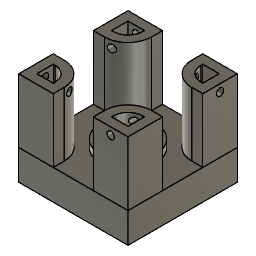
pince (Autodesk Fusion 360 archive; units mm, degrees)
design "pince_v01_structure"
part number: 2026-02-12-14-10-12-234
Autodesk Fusion 360 part; units mm, degrees
sketch "Esquisse1" plane through (0, 0, 0) normal (0, 0, 1) x (1, 0, 0)
  line L0 (30, 30) -> (-30, 30)
  line L1 (-30, 30) -> (-30, -30)
  line L2 (-30, -30) -> (30, -30)
  line L3 (30, -30) -> (30, 30)
  constraint horizontal L0
  constraint vertical L1
  constraint horizontal L2
  constraint vertical L3
extrude "Extrusion1" add sketch "Esquisse1" along normal blind 5 makes body 1
sketch "Esquisse3" plane through (0, 0, 5) normal (0, 0, 1) x (-1, 0, 0)
  line L0 (-30, 30) -> (-30, -30)
  line L1 (-30, -30) -> (30, -30)
  line L2 (30, -30) -> (30, 30)
  line L3 (30, 30) -> (-30, 30)
  circle A0 centre (0, 0) radius 3.5
  circle A1 centre (0, 0) radius 15
  dimension "d12" = 7
  dimension "d15" = 30
  constraint coincident A0.centre A1.centre
  measures "d12" diameter of A0
  measures "d15" diameter of A1
extrude "Extrusion2" add sketch "Esquisse3" along normal blind 4 contours A1 bodies 1
sketch "Esquisse4" plane through (0, 0, 5) normal (0, 0, 1) x (-1, 0, 0)
  line L0 (-30, 30) -> (-30, -30)
  line L1 (-30, -30) -> (30, -30)
  line L2 (30, -30) -> (30, 30)
  line L3 (30, 30) -> (-30, 30)
  circle A0 centre (0, 0) radius 15
  arc A1 (-24, 11) -> (-11, 24) centre (-24, 24) ccw
  line L4 (-11, 24) -> (-30, 24)
  line L5 (-30, 24) -> (-30, 30)
  line L6 (-30, 30) -> (-11, 30)
  line L7 (-11, 30) -> (-11, 24)
  line L8 (-30, 30) -> (-24, 30)
  line L9 (-24, 30) -> (-24, 11)
  line L10 (-24, 11) -> (-30, 11)
  line L11 (-30, 11) -> (-30, 30)
  constraint horizontal L4
  constraint vertical L5
  constraint horizontal L6
  constraint vertical L7
  constraint coincident L0.start L3.end
  constraint horizontal L8
  constraint vertical L9
  constraint horizontal L10
  constraint vertical L11
extrude "Extrusion3" add sketch "Esquisse4" along normal up to surface (70 mm away) contours L0 L3 L4 L5 L6 L8 L9 L11 | L0 L4 L9 L10 L11 | L3 L4 L6 L7 L9 | A1 L4 L9 bodies 1
sketch "Esquisse5" plane through (0, 0, 0) normal (0, 1, 0) x (1, 0, 0)
  line L0 (-30, 0) -> (30, 0)
  line L1 (30, 0) -> (30, 9.0556)
  line L2 (30, 19.372) -> (-30, 19.372)
  line L3 (-30, 9.0556) -> (-30, 0)
  circle A0 centre (0, 36) radius 34.3
  arc A1 (-25.7143, 10.8052) -> (25.7143, 10.8052) centre (0, 36) ccw
  arc A2 (-25.7143, 10.8052) -> (-30, 9.0556) centre (-27.5, 9.0556) ccw
  arc A3 (30, 9.0556) -> (25.7143, 10.8052) centre (27.5, 9.0556) ccw
  line L4 (-30, 7.5) -> (-27.5, 7.5)
  line L5 (-27.5, 7.5) -> (-27.5, 11.5556)
  line L6 (-27.5, 11.5556) -> (-30, 11.5556)
  line L7 (-30, 11.5556) -> (-30, 7.5)
  point P0 (-30, 0)
  dimension "d80" = 36
  dimension "d81" = 2.5
  dimension "d82" = 2.5
  dimension "d83" = 2.5
  constraint horizontal L0
  constraint vertical L1
  constraint horizontal L2
  constraint vertical L3
  constraint coincident L2.start A0
  constraint coincident P0 L0.start
  constraint coincident A0.centre A1.centre
  constraint tangent A1 A2
  constraint tangent L3 A2
  constraint tangent A1 A3
  constraint tangent L1 A3
  constraint horizontal L4
  constraint vertical L5
  constraint horizontal L6
  constraint vertical L7
  constraint coincident L3 L4.start
  measures "d80" radius of A1
  measures "d81" radius of A2
  measures "d82" radius of A3
  measures "d83" distance of L4.start L4.end
revolve "Révolution2" add sketch "Esquisse5" angle 360 about axis through (0, 0, -205.75) along (0, 0, 1) contours L0 L3 A1 A2 L4 L5 | L3 A2 L4 L5 L7 | A2 L6 L7 bodies 1
extrude "Extrusion4" add 4 faces at (-24.1061, -24.1061, 0) (24.1061, -24.1061, 0) (24.1061, 24.1061, 0) (-24.1061, 24.1061, 0) along direction (0, 0, -1) up to surface end surface through (0, 0, -11.5556) normal (0, 0, -1) offset 0 on bodies 1 bodies 1
extrude "Extrusion5" cut 1 faces at (28, -17.3333, 75) along direction (0, 0, -1) blind 35 on bodies 1 bodies 1
sketch "Esquisse7" plane through (0, 0, 40) normal (0, 0, 1) x (-1, 0, 0)
  line L0 (-30, 11) -> (-24, 11)
  arc A0 (-24, 11) -> (-11, 24) centre (-24, 24) ccw
  line L1 (-11, 24) -> (-11, 30)
  line L2 (-11, 30) -> (-30, 30)
  line L3 (-30, 30) -> (-30, 11)
  line L4 (-16, 24) -> (-16, 25)
  line L5 (-16, 25) -> (-25, 25)
  line L6 (-25, 25) -> (-25, 16)
  line L7 (-25, 16) -> (-24, 16)
  arc A1 (-24, 16) -> (-16, 24) centre (-24, 24) ccw
  dimension "d157" = -5
extrude "Extrusion7" cut sketch "Esquisse7" against normal blind 10 contours L4 L5 L6 L7 A1 bodies 1
pattern_circular "Réseau C2" count 4 over 360 about axis through (0, 0, -205.75) along (0, 0, 1) of bodies 1 makes body 2 at (30, 23.6667, 11.1481) makes body 3 at (-23.6667, 30, 11.1481) makes body 4 at (-30, -23.6667, 11.1481)
sketch "Esquisse8" plane through (0, -30, 0) normal (0, -1, 0) x (1, 0, 0)
  line L0 (30, 40) -> (11, 40)
  line L1 (11, 40) -> (11, 5)
  line L2 (11, 5) -> (-30, 5)
  line L3 (-30, 5) -> (-30, -11.5556)
  line L4 (-30, -11.5556) -> (30, -11.5556)
  line L5 (30, -11.5556) -> (30, 40)
  line L6 (11, 40) -> (30, 40)
  line L7 (30, 40) -> (30, 36)
  line L8 (30, 36) -> (11, 36)
  line L9 (11, 36) -> (11, 40)
  circle A0 centre (20.5, 36) radius 2
  dimension "d3" = 4
  dimension "d4" = 4
  constraint horizontal L6
  constraint vertical L7
  constraint horizontal L8
  constraint vertical L9
  constraint coincident L0.end L1.start
  constraint midpoint L8 A0.centre
  measures "d3" distance of L0.end L8.end
  measures "d4" diameter of A0
extrude "Extrusion8" cut sketch "Esquisse8" against normal up to surface (19 mm away) contours L8 A0 | L8 A0 bodies 1
sketch "Esquisse9" plane through (-30, 0, 0) normal (-1, 0, 0) x (0, -1, 0)
  line L0 (30, 40) -> (11, 40)
  line L1 (11, 40) -> (11, 5)
  line L2 (11, 5) -> (-30, 5)
  line L3 (-30, 5) -> (-30, -11.5556)
  line L4 (-30, -11.5556) -> (30, -11.5556)
  line L5 (30, -11.5556) -> (30, 40)
  line L6 (30, 40) -> (11, 40)
  line L7 (30, 40) -> (30, 36)
  line L8 (30, 36) -> (11, 36)
  line L9 (11, 36) -> (11, 40)
  circle A0 centre (20.5, 36) radius 2
  line L10 (11, 40) -> (30, 40)
  dimension "d7" = 4
  dimension "d8" = 4
  constraint horizontal L10
  constraint vertical L7
  constraint horizontal L8
  constraint vertical L9
  constraint coincident L0.end L1.start
  constraint midpoint A0.centre L8
  measures "d7" distance of L0.end L8.end
  measures "d8" diameter of A0
sketch "Esquisse10" plane through (0, 30, 0) normal (0, 1, 0) x (-1, 0, 0)
  line L0 (30, 40) -> (11, 40)
  line L1 (11, 40) -> (11, 5)
  line L2 (11, 5) -> (-30, 5)
  line L3 (-30, 5) -> (-30, -11.5556)
  line L4 (-30, -11.5556) -> (30, -11.5556)
  line L5 (30, -11.5556) -> (30, 40)
  line L6 (30, 40) -> (11, 40)
  line L7 (30, 40) -> (30, 36)
  line L8 (30, 36) -> (11, 36)
  line L9 (11, 36) -> (11, 40)
  circle A0 centre (20.5, 36) radius 2
  line L10 (11, 40) -> (30, 40)
  dimension "d9" = 4
  dimension "d10" = 4
  constraint horizontal L10
  constraint vertical L7
  constraint horizontal L8
  constraint vertical L9
  constraint coincident L0.end L1.start
  constraint midpoint A0.centre L8
  measures "d9" distance of L0.end L8.end
  measures "d10" diameter of A0
sketch "Esquisse11" plane through (30, 0, 0) normal (1, 0, 0) x (0, 1, 0)
  line L0 (30, 40) -> (11, 40)
  line L1 (11, 40) -> (11, 5)
  line L2 (11, 5) -> (-30, 5)
  line L3 (-30, 5) -> (-30, -11.5556)
  line L4 (-30, -11.5556) -> (30, -11.5556)
  line L5 (30, -11.5556) -> (30, 40)
  line L6 (30, 40) -> (11, 40)
  line L7 (30, 40) -> (30, 36)
  line L8 (30, 36) -> (11, 36)
  line L9 (11, 36) -> (11, 40)
  circle A0 centre (20.5, 36) radius 2
  line L10 (11, 40) -> (30, 40)
  dimension "d11" = 4
  dimension "d16" = 4
  constraint horizontal L10
  constraint vertical L7
  constraint horizontal L8
  constraint vertical L9
  constraint coincident L0.end L1.start
  constraint midpoint A0.centre L8
  measures "d11" distance of L0.end L8.end
  measures "d16" diameter of A0
extrude "Extrusion9" cut sketch "Esquisse9" against normal up to surface (19 mm away) contours L8 A0 | L8 A0 bodies 4
extrude "Extrusion10" cut sketch "Esquisse10" against normal up to surface (19 mm away) contours L8 A0 | L8 A0 bodies 3
extrude "Extrusion11" cut sketch "Esquisse11" against normal up to surface (19 mm away) contours L8 A0 | L8 A0 bodies 2

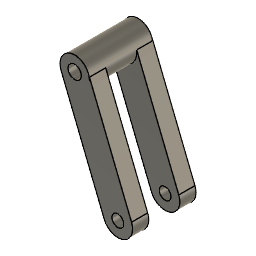
design "pince_v01_second_arm"
part number: 2026-02-12-19-33-38-702
Autodesk Fusion 360 part; units mm, degrees
sketch "Esquisse1" plane through (0, -10.5, 0) normal (0, 1, 0) x (-1, 0, 0)
  circle A0 centre (-25, 50) radius 2
  line L0 (-30, 56) -> (-30, 40)
  line L1 (-30, 40) -> (-18, 40)
  line L2 (-18, 40) -> (-18, 56)
  line L3 (-18, 56) -> (-30, 56)
  circle A1 centre (-25, 50) radius 2.25
  circle A2 centre (-25, 50) radius 5
  circle A3 centre (-39.6076, 13.6901) radius 5
  circle A4 centre (-39.6076, 13.6901) radius 2
  line L4 (-25, 50) -> (-39.6076, 13.6901)
  line L5 (-29.6387, 51.8662) -> (-44.2463, 15.5563)
  line L6 (-20.3613, 48.1338) -> (-34.9689, 11.824)
  point P0 (-22.75, 50.0115)
  point P1 (-39.6076, 13.6901)
  dimension "d228" = 10
  dimension "d229" = 10
  dimension "d230" = 4
  constraint concentric A0 A1
  constraint coincident A1 P0
  constraint concentric A1 A2
  constraint coincident P1 A3.centre
  constraint concentric A3 A4
  constraint coincident A0.centre A1.centre
  measures "d228" diameter of A2
  measures "d229" diameter of A3
  measures "d230" diameter of A4
extrude "Extrusion1" add sketch "Esquisse1" along normal blind 5.25 contours L0 L1 A3 L4 L5 | L0 L1 A2 L4 | A3 | L1 A2 L4 L6 | L1 A3 L4 L6
extrude "Extrusion2" add sketch "Esquisse1" along normal blind 10.5 contours A2
move_body "Déplacer1" bodies 1 to x (1, 0, 0) y (0, 1, 0) z (0, 0, 1) at (0, 0.25, 0)
extrude "Extrusion3" cut 1 faces at (31.7625, -10.25, 37.8971) along direction (0, 1, 0) blind 0.25
extrude "Extrusion4" cut 1 faces at (20.9437, 0.25, 50.3602) along direction (0, -1, 0) blind 0.25
mirror "Symétrie miroir1" about plane through (0, 0, 0) normal (0, 1, 0) of bodies 1 merged
extrude "Extrusion5" add 1 faces at (31.7625, -10, 37.8971) along direction (0, -1, 0) blind 0.25
extrude "Extrusion6" cut 1 faces at (37.5808, -5, 25.9737) along direction (0, -1, 0) blind 0.25
extrude "Extrusion7" add 1 faces at (31.7625, 10, 37.8971) along direction (0, 1, 0) blind 0.25
extrude "Extrusion8" cut 1 faces at (37.5808, 5, 25.9737) along direction (0, 1, 0) blind 0.25
extrude "Extrusion9" add 1 faces at (31.7625, -10.25, 37.8971) along direction (0, -1, 0) blind 0.5
extrude "Extrusion10" add 1 faces at (31.7625, 10.25, 37.8971) along direction (0, 1, 0) blind 0.5

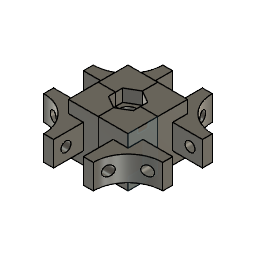
design "pince_v02_mobile"
part number: 2026-02-11-00-55-34-916
Autodesk Fusion 360 part; units mm, degrees
sketch "Esquisse1" plane through (0, 0, 5) normal (0, 0, 1) x (-1, 0, 0)
  line L0 (0, 0, 20) -> (-15, 0, 20)
  line L1 (-15, 0, 20) -> (-15, 15, 20)
  line L2 (-15, 15, 20) -> (0, 15, 20)
  line L3 (0, 15, 20) -> (0, 0, 20)
  dimension "d16" = 15
  dimension "d17" = 15
extrude "Extrusion1" add sketch "Esquisse1" along normal blind 20 contours L0 L1 L2 L3 in plane through (0, 0, 25) normal (0, 0, 1) makes body 1
sketch "Esquisse2" plane through (0, 0, 0) normal (-1, 0, 0) x (0, -1, 0)
  line L0 (0, 25) -> (15, 25)
  line L1 (15, 25) -> (15, 45)
  line L2 (15, 45) -> (0, 45)
  line L3 (0, 45) -> (0, 25)
  line L4 (0, 35) -> (8, 35)
  line L5 (8, 35) -> (8, 38)
  line L6 (8, 38) -> (0, 38)
  line L7 (0, 38) -> (0, 35)
  dimension "d20" = 8
  dimension "d21" = 3
  constraint horizontal L4
  constraint vertical L5
  constraint horizontal L6
  constraint vertical L7
  constraint midpoint L3 L4.start
  measures "d20" distance of L4.start L4.end
  measures "d21" distance of L4.start L6.end
extrude "Extrusion2" cut sketch "Esquisse2" against normal blind 8 contours L3 L4 L5 L6 L7 bodies 1
sketch "Esquisse3" plane through (0, 0, 45) normal (0, 0, 1) x (-1, 0, 0)
  line L0 (0, 15) -> (-15, 15)
  line L1 (-15, 15) -> (-15, 0)
  line L2 (-15, 0) -> (0, 0)
  line L3 (0, 0) -> (0, 15)
  circle A0 centre (0, 0) radius 3.5
  dimension "d24" = 7
  constraint coincident L2.end L3.start
  measures "d24" diameter of A0
extrude "Extrusion3" cut sketch "Esquisse3" against normal blind 20 contours L2 L3 A0 picked at (-1.8632, 1.3948) bodies 1
extrude "Extrusion4" cut 1 faces at (6.3148, -3.2974, 35) along direction (0, 0, -1) blind 3 on bodies 1 bodies 1
extrude "Extrusion5" cut 1 faces at (10, -15, 38.3333) along direction (0, 1, 0) blind 3 on bodies 1 bodies 1
extrude "Extrusion6" cut 1 faces at (15, -4, 38.3333) along direction (-1, 0, 0) blind 3 on bodies 1 bodies 1
sketch "Esquisse4" plane through (0, 0, 0) normal (-1, 0, 0) x (0, -1, 0)
  line L0 (12, 25) -> (12, 45)
  line L1 (12, 45) -> (3.5, 45)
  line L2 (3.5, 45) -> (3.5, 38)
  line L3 (3.5, 38) -> (8, 38)
  line L4 (8, 38) -> (8, 32)
  line L5 (8, 32) -> (3.5, 32)
  line L6 (3.5, 32) -> (3.5, 25)
  line L7 (3.5, 25) -> (12, 25)
  circle A0 centre (7.75, 41.5) radius 2
  circle A1 centre (7.75, 28.5) radius 2
  dimension "d33" = 4
  dimension "d34" = 4
  measures "d33" diameter of A0
  measures "d34" diameter of A1
extrude "Extrusion7" cut sketch "Esquisse4" against normal blind 6 contours A0 | A1 bodies 1
sketch "Esquisse5" plane through (0, 0, 0) normal (0, 1, 0) x (-1, 0, 0)
  line L0 (-12, 45) -> (-12, 25)
  line L1 (-12, 25) -> (-3.5, 25)
  line L2 (-3.5, 25) -> (-3.5, 32)
  line L3 (-3.5, 32) -> (-8, 32)
  line L4 (-8, 32) -> (-8, 38)
  line L5 (-8, 38) -> (-3.5, 38)
  line L6 (-3.5, 38) -> (-3.5, 45)
  line L7 (-3.5, 45) -> (-12, 45)
  circle A0 centre (-7.75, 41.5) radius 1.75
  circle A1 centre (-7.75, 28.5) radius 1.75
  dimension "d37" = 3.5
  dimension "d38" = 3.5
  measures "d37" diameter of A0
  measures "d38" diameter of A1
extrude "Extrusion8" add sketch "Esquisse5" along normal blind 4 contours A0 | A1 bodies 1
extrude "Extrusion9" add 2 faces at (6, -7.5064, 28.7863) (6, -7.1494, 41.2107) along direction (-1, 0, 0) blind 1 on bodies 1 bodies 1
sketch "Esquisse6" plane through (0, 0, 0) normal (0, 1, 0) x (-1, 0, 0)
  circle A0 centre (-7.75, 28.5) radius 1.75
  circle A1 centre (-7.75, 41.5) radius 1.75
  line L0 (-12, 45) -> (-12, 25)
  line L1 (-12, 25) -> (-3.5, 25)
  line L2 (-3.5, 25) -> (-3.5, 32)
  line L3 (-3.5, 32) -> (-8, 32)
  line L4 (-8, 32) -> (-8, 38)
  line L5 (-8, 38) -> (-3.5, 38)
  line L6 (-3.5, 38) -> (-3.5, 45)
  line L7 (-3.5, 45) -> (-12, 45)
  line L8 (-12, 45) -> (-24, 45)
  line L9 (-24, 45) -> (-24, 25)
  line L10 (-24, 25) -> (-12, 25)
  line L11 (-12, 25) -> (-12, 45)
  line L12 (-24, 40) -> (-14, 40)
  line L13 (-14, 40) -> (-14, 30)
  line L14 (-14, 30) -> (-24, 30)
  line L15 (-24, 30) -> (-24, 40)
  circle A2 centre (-19, 35) radius 2
  line L16 (-14, 40) -> (-12, 40)
  line L17 (-12, 40) -> (-12, 30)
  line L18 (-12, 30) -> (-14, 30)
  line L19 (-14, 30) -> (-14, 40)
  dimension "d43" = 12
  dimension "d44" = 10
  dimension "d45" = 4
  constraint horizontal L8
  constraint vertical L9
  constraint horizontal L10
  constraint vertical L11
  constraint coincident L0.start L7.end
  constraint horizontal L12
  constraint vertical L13
  constraint horizontal L14
  constraint vertical L15
  constraint coincident L9 L12.start
  constraint horizontal L16
  constraint vertical L17
  constraint horizontal L18
  constraint vertical L19
  constraint coincident L11 L17.end
  measures "d43" distance of L0.start L8.end
  measures "d44" distance of L12.start L12.end
  measures "d45" diameter of A2
extrude "Extrusion10" add sketch "Esquisse6" against normal blind 10 contours L0 L11 L13 L16 L17 L18 L19 | L9 L12 L13 L14 L15 L19 bodies 1
extrude "Extrusion11" cut sketch "Esquisse6" against normal blind 6 contours L0 L11 L13 L16 L17 L18 L19 | L9 L12 L13 L14 L15 L19 bodies 1
sketch "Esquisse7" plane through (0, 0, 0) normal (-1, 0, 0) x (0, -1, 0)
  circle A0 centre (7.75, 41.5) radius 2
  circle A1 centre (7.75, 28.5) radius 2
  line L0 (12, 25) -> (12, 45)
  line L1 (12, 45) -> (3.5, 45)
  line L2 (3.5, 45) -> (3.5, 38)
  line L3 (3.5, 38) -> (8, 38)
  line L4 (8, 38) -> (8, 32)
  line L5 (8, 32) -> (3.5, 32)
  line L6 (3.5, 32) -> (3.5, 25)
  line L7 (3.5, 25) -> (12, 25)
  line L8 (12, 45) -> (24, 45)
  line L9 (24, 45) -> (24, 25)
  line L10 (24, 25) -> (12, 25)
  line L11 (12, 25) -> (12, 45)
  line L12 (24, 40) -> (14, 40)
  line L13 (14, 40) -> (14, 30)
  line L14 (14, 30) -> (24, 30)
  line L15 (24, 30) -> (24, 40)
  line L16 (14, 40) -> (12, 40)
  line L17 (12, 40) -> (12, 30)
  line L18 (12, 30) -> (14, 30)
  line L19 (14, 30) -> (14, 40)
  circle A2 centre (19, 35) radius 2
  dimension "d50" = 12
  dimension "d51" = 10
  dimension "d52" = 10
  dimension "d53" = 4
  constraint horizontal L8
  constraint vertical L9
  constraint horizontal L10
  constraint vertical L11
  constraint coincident L0.end L1.start
  constraint horizontal L12
  constraint vertical L13
  constraint horizontal L14
  constraint vertical L15
  constraint horizontal L16
  constraint vertical L17
  constraint horizontal L18
  constraint vertical L19
  constraint coincident L11 L17.end
  measures "d50" distance of L0.end L8.end
  measures "d51" distance of L12.start L12.end
  measures "d52" distance of L12.start L14.end
  measures "d53" diameter of A2
extrude "Extrusion12" add sketch "Esquisse7" against normal blind 10 contours L0 L11 L13 L16 L17 L18 L19 | L9 L12 L13 L14 L15 L19 bodies 1
extrude "Extrusion13" cut sketch "Esquisse7" against normal blind 6 contours L0 L11 L13 L16 L17 L18 L19 | L9 L12 L13 L14 L15 L19 bodies 1
sketch "Esquisse8" plane through (0, 0, 30) normal (0, 0, -1) x (1, 0, 0)
  line L0 (12, 6) -> (24, 6)
  line L1 (24, 6) -> (24, 10)
  line L2 (24, 10) -> (12, 10)
  line L3 (12, 10) -> (12, 6)
  line L4 (10, 24) -> (24, 24)
  line L5 (24, 24) -> (24, 10)
  line L6 (24, 10) -> (10, 10)
  line L7 (10, 10) -> (10, 24)
  circle A0 centre (24, 24) radius 14
  point P0 (10, 24)
  constraint horizontal L4
  constraint vertical L5
  constraint horizontal L6
  constraint vertical L7
  constraint coincident L1.end L2.start
  constraint coincident P0 L4.start
  constraint coincident L4.end L5.start
  constraint coincident L1.end A0
extrude "Extrusion14" add sketch "Esquisse8" against normal blind 10 contours L2 L6 L7 A0 bodies 1
extrude "Extrusion15" cut 1 faces at (19.4157, -10, 35.5212) along direction (0, 1, 0) up to surface end surface at (23.3339, -10.0159, 36.6667) on bodies 1 bodies 1
extrude "Extrusion16" cut 1 faces at (10, -19.5583, 34.7238) along direction (-1, 0, 0) up to surface end surface at (22.9927, -10.0363, 35.0226) on bodies 1 bodies 1
sketch "Esquisse9" plane through (12, 0, 0) normal (1, 0, 0) x (0, 1, 0)
  line L0 (-6, 30) -> (-12, 30)
  line L1 (-12, 30) -> (-12, 25)
  line L2 (-12, 25) -> (0, 25)
  line L3 (0, 25) -> (0, 45)
  line L4 (0, 45) -> (-12, 45)
  line L5 (-12, 45) -> (-12, 40)
  line L6 (-12, 40) -> (-6, 40)
  line L7 (-6, 40) -> (-6, 30)
  line L8 (-6, 45) -> (-4, 45)
  line L9 (-4, 45) -> (-4, 43)
  line L10 (-4, 43) -> (-6, 43)
  line L11 (-6, 43) -> (-6, 45)
  line L12 (-6, 43) -> (-6, 45)
  line L13 (-6, 45) -> (-8, 45)
  line L14 (-8, 43) -> (-6, 43)
  line L15 (-8, 45) -> (-8, 43)
  dimension "d64" = 2
  dimension "d65" = 2
  constraint horizontal L8
  constraint vertical L9
  constraint horizontal L10
  constraint vertical L11
  constraint midpoint L4 L8.start
  constraint symmetric L8.start L11 L12.end
  constraint symmetric L8.end L11 L13.end
  constraint symmetric L9.end L11 L14.start
  constraint symmetric L10.end L11 L12.start
  measures "d64" distance of L8.start L8.end
  measures "d65" distance of L8.start L10.end
extrude "Extrusion17" add sketch "Esquisse9" along normal blind 1 contours L4 L11 L12 L13 L14 L15 | L4 L8 L9 L10 L11 L12 bodies 1
sketch "Esquisse10" plane through (0, -4, 0) normal (0, 1, 0) x (-1, 0, 0)
  line L0 (-12, 43) -> (-12, 45)
  line L1 (-12, 45) -> (-13, 45)
  line L2 (-13, 45) -> (-13, 43)
  line L3 (-13, 43) -> (-12, 43)
  line L4 (-13, 43) -> (-12, 45)
  constraint coincident L2.end L3.start
  constraint coincident L0.end L1.start
extrude "Extrusion18" cut sketch "Esquisse10" against normal blind 4 contours L1 L2 L4 bodies 1
sketch "Esquisse11" plane through (12, 0, 0) normal (1, 0, 0) x (0, 1, 0)
  line L0 (-8, 43) -> (-8, 45)
  line L1 (-8, 45) -> (-12, 45)
  line L2 (-12, 45) -> (-12, 40)
  line L3 (-12, 40) -> (-6, 40)
  line L4 (-6, 40) -> (-6, 30)
  line L5 (-6, 30) -> (-12, 30)
  line L6 (-12, 30) -> (-12, 25)
  line L7 (-12, 25) -> (0, 25)
  line L8 (0, 25) -> (0, 45)
  line L9 (0, 45) -> (-4, 45)
  line L10 (-4, 45) -> (-4, 43)
  line L11 (-4, 43) -> (-8, 43)
sketch "Esquisse12" plane through (0, -12, 0) normal (0, -1, 0) x (1, 0, 0)
  line L0 (12, 30) -> (6, 30)
  line L1 (6, 30) -> (6, 40)
  line L2 (6, 40) -> (12, 40)
  line L3 (12, 40) -> (12, 45)
  line L4 (12, 45) -> (0, 45)
  line L5 (0, 45) -> (0, 25)
  line L6 (0, 25) -> (12, 25)
  line L7 (12, 25) -> (12, 30)
  line L8 (6, 25) -> (8, 25)
  line L9 (8, 25) -> (8, 27)
  line L10 (8, 27) -> (6, 27)
  line L11 (6, 27) -> (6, 25)
  line L12 (6, 27) -> (6, 25)
  line L13 (6, 25) -> (4, 25)
  line L14 (4, 27) -> (6, 27)
  line L15 (4, 25) -> (4, 27)
  dimension "d70" = 2
  dimension "d71" = 2
  constraint horizontal L8
  constraint vertical L9
  constraint horizontal L10
  constraint vertical L11
  constraint midpoint L6 L8.start
  constraint symmetric L8.start L11 L12.end
  constraint symmetric L8.end L11 L13.end
  constraint symmetric L9.end L11 L14.start
  constraint symmetric L10.end L11 L12.start
  measures "d70" distance of L8.start L8.end
  measures "d71" distance of L8.start L10.end
extrude "Extrusion19" add sketch "Esquisse12" along normal blind 1 contours L6 L8 L9 L10 L11 L12 | L6 L11 L12 L13 L14 L15 bodies 1
sketch "Esquisse13" plane through (4, 0, 0) normal (-1, 0, 0) x (0, -1, 0)
  line L0 (12, 27) -> (12, 25)
  line L1 (12, 25) -> (13, 25)
  line L2 (13, 25) -> (13, 27)
  line L3 (13, 27) -> (12, 27)
  line L4 (12, 25) -> (12.1, 25.2)
  line L5 (12.1, 25.2) -> (13, 27)
  constraint coincident L0.end L1.start
  constraint coincident L2.end L3.start
extrude "Extrusion20" cut sketch "Esquisse13" against normal blind 4 contours L1 L2 L4 L5 bodies 1
extrude "Extrusion21" cut 1 faces at (12.3333, -4, 43.6667) along direction (0, -1, 0) blind 4 on bodies 1 bodies 1
extrude "Extrusion22" add 2 faces at (5, -7.1494, 41.2107) (5, -7.5064, 28.7863) along direction (-1, 0, 0) blind 5 on bodies 1 bodies 1
extrude "Extrusion23" cut 2 faces at (7.8798, 4, 42.0687) (8.0417, 4, 29.0052) along direction (0, -1, 0) blind 4 on bodies 1 bodies 1
extrude "Extrusion24" cut 1 faces at (4, -12.3667, 26.4) along direction (1, 0, 0) blind 4 on bodies 1 bodies 1
extrude "Extrusion25" add 1 faces at (6.3148, -3.2974, 38) along direction (0, 0, -1) blind 6 on bodies 1 bodies 1
pattern_circular "Réseau C1" count 4 over 360 about axis through (0, 0, 1.75) along (0, 0, 1) of bodies 1 makes body 2 at (10.0363, 22.9927, 35.0226) makes body 3 at (-22.9927, 10.0363, 35.0226) makes body 4 at (-10.0363, -22.9927, 35.0226)
sketch "Esquisse14" plane through (0, 0, 45) normal (0, 0, 1) x (-1, 0, 0)
  line L0 (-12, -12) -> (0, -12)
  line L1 (0, -12) -> (0, -3.5)
  arc A0 (-3.5, 0) -> (0, -3.5) centre (0, 0) ccw
  line L2 (-3.5, 0) -> (-12, 0)
  line L3 (-12, 0) -> (-12, -12)
  line L4 (0, 5.8) -> (-5.0229, 2.9)
  line L5 (-5.0229, 2.9) -> (-5.0229, -2.9)
  line L6 (-5.0229, -2.9) -> (0, -5.8)
  line L7 (0, -5.8) -> (5.0229, -2.9)
  line L8 (5.0229, -2.9) -> (5.0229, 2.9)
  line L9 (5.0229, 2.9) -> (0, 5.8)
  line L10 (0, 3.5) -> (0, 12)
  dimension "d13" = 5.8
  constraint coincident A0.centre origin
  constraint coincident L4.start L10
  measures "d13" distance of L4.start A0.centre
extrude "Extrusion26" cut sketch "Esquisse14" against normal blind 5 contours L1 A0 L2 L5 L6 | L1 A0 L2 L4 L5 L7 L8 L9 bodies 1 2 3 4
sketch "Esquisse15" plane through (0, 0, 25) normal (0, 0, -1) x (1, 0, 0)
  line L0 (12, 12) -> (0, 12)
  line L1 (0, 12) -> (0, 3.5)
  arc A0 (3.5, 0) -> (0, 3.5) centre (0, 0) ccw
  line L2 (3.5, 0) -> (12, 0)
  line L3 (12, 0) -> (12, 12)
  line L4 (0, 5.8) -> (-5.0229, 2.9)
  line L5 (-5.0229, 2.9) -> (-5.0229, -2.9)
  line L6 (-5.0229, -2.9) -> (0, -5.8)
  line L7 (0, -5.8) -> (5.0229, -2.9)
  line L8 (5.0229, -2.9) -> (5.0229, 2.9)
  line L9 (5.0229, 2.9) -> (0, 5.8)
  dimension "d76" = 5.8
  constraint coincident A0.centre origin
  measures "d76" distance of L4.start A0.centre
extrude "Extrusion27" cut sketch "Esquisse15" against normal blind 5 contours L1 A0 L2 L8 L9 | L1 A0 L2 L4 L5 L6 L7 L8 bodies 1 2 3 4
